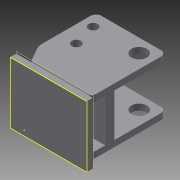
# Autodesk Inventor part: sketss
Saved by Autodesk Inventor 2014 SP2 (Build 180246200, 246)
## iProperties
Created: 2019-06-25
Part Number: sketss
Material: Generic
Document SubType Name: Modeling
Designer: USER PC
Density: 1 g/cm^3
Appearance: Default
Author: USER PC
Autodesk Inventor part; units mm, degrees
ref_plane "YZ Plane" through (0, 0, 0) normal (1, 0, 0) x (0, 1, 0)
ref_plane "XY Plane" through (0, 0, 0) normal (0, 0, 1) x (1, 0, 0)
sketch "Sketch1" plane through (0, 0, 0) normal (0, 0, 1) x (1, 0, 0)
  circle A0 centre (0, 0) radius 15
  circle A1 centre (150, 0) radius 25
  line L0 (-35, 45) -> (-35, -144.3782)
  circle A2 centre (43.934, -106.066) radius 15
  circle A3 centre (20.0962, -75) radius 15
  line L1 (195, 45) -> (-35, 45)
  line L2 (195, -205) -> (0, -205)
  line L3 (195, -205) -> (195, 45)
  line L4 (0, -205) -> (-35, -144.3782)
  line L5 (0, -205) -> (70, -205) construction
  dimension "d22" = 230
  dimension "d23" = 120
  constraints: 12 end point, 4 centre point, 1 coincident, 1 equal length, 1 horizontal, 1 parallel, 1 perpendicular
  measures "d22" distance of L1.start L0.start
  measures "d23" angle of L5 L4
extrude "Extrusion1" add sketch "Sketch1" along normal blind 180
fillet "Fillet1" radius 50 1 edges at (-35, -144.3782, 90)
fillet "Fillet2" radius 20 1 edges at (-35, 45, 90)
fillet "Fillet3" radius 20 1 edges at (195, 45, 90)
fillet "Fillet4" radius 20 1 edges at (195, -205, 90)
fillet "Fillet5" radius 20 1 edges at (0, -205, 90)
sketch "Sketch2" plane through (-35, -130.9808, 0) normal (-1, 0, 0) x (0, 0, 1)
  line L0 (0, 155.9808) -> (180, 155.9808) projected
  line L1 (0, 155.9808) -> (0, 0) projected
  line L2 (180, 155.9808) -> (180, 0) projected
  line L3 (0, 175) -> (0, -75)
  line L4 (0, -75) -> (20, -75)
  line L5 (20, -75) -> (20, -25)
  line L6 (20, -25) -> (160, -25)
  line L7 (160, -25) -> (160, -75)
  line L8 (160, -75) -> (180, -75)
  line L9 (180, -75) -> (180, 175)
  line L10 (180, 175) -> (160, 175)
  line L11 (160, 175) -> (160, 5)
  line L12 (160, 5) -> (20, 5)
  line L13 (20, 5) -> (20, 175)
  line L14 (20, 175) -> (0, 175)
  point P0 (0, 130.9808)
  dimension "d31" = 250
  dimension "d32" = 20
  dimension "d33" = 50
  dimension "d34" = 140
  dimension "d35" = 170
  constraints: 24 end point, 8 parallel, 3 perpendicular, 1 collinear, 1 point on line
  measures "d31" distance of L3.start L3.end
  measures "d32" distance of L3.end L4.end
  measures "d33" distance of L4.end L5.end
  measures "d34" distance of L5.end L6.end
  measures "d35" distance of L10.end L11.end
extrude "Extrusion2" cut sketch "Sketch2" against normal blind 230 contours L3 L14 L13 L0 | L0 L13 L12 L11 L2 L9 L8 L7 L6 L5 L4 L3 L1 | L11 L10 L9 L0 keep common part
sketch "Sketch3" plane through (0, 0, 180) normal (0, 0, 1) x (1, 0, 0)
  circle A0 centre (43.934, -106.066) radius 15 projected
  circle A1 centre (43.934, -106.066) radius 15
  constraints: 1 centre point, 1 coincident, 1 concentric
extrude "Extrusion3" add sketch "Sketch3" against normal blind 20
sketch "Sketch4" plane through (0, 0, 0) normal (0, 0, -1) x (-1, 0, 0)
  circle A0 centre (-43.934, -106.066) radius 15 projected
  circle A1 centre (-43.934, -106.066) radius 15
  constraints: 1 centre point, 1 coincident, 1 concentric
extrude "Extrusion4" add sketch "Sketch4" against normal blind 20
ref_plane "Work Plane1" through (175, -205, 20) normal (0, 1, 0) x (-1, 0, 0)
sketch "Sketch6" plane through (175, -205, 20) normal (0, 1, 0) x (-1, 0, 0)
  line L0 (-19.2308, -36.5385) -> (221.1538, -36.5385)
  line L1 (221.1538, -36.5385) -> (221.1538, 163.4615)
  line L2 (221.1538, 163.4615) -> (-28.8462, 163.4615)
  line L3 (-28.8462, 163.4615) -> (-28.8462, -36.5385)
  line L4 (-28.8462, -36.5385) -> (-19.2308, -36.5385)
  point P0 (175, -20)
  dimension "d55" = 250
  dimension "d56" = 200
  constraints: 10 end point, 2 perpendicular, 1 parallel
  measures "d55" distance between parallel lines of L3 L1
  measures "d56" distance of L0.end L1.end
extrude "Extrusion6" add sketch "Sketch6" against normal blind 20
sketch "Sketch7" plane through (175, -225, 20) normal (0, -1, 0) x (1, 0, 0)
  line L0 (-221.1538, -36.5385) -> (28.8462, -36.5385) projected
  line L1 (28.8462, -36.5385) -> (28.8462, 163.4615) projected
  line L2 (28.8462, 163.4615) -> (-221.1538, 163.4615) projected
  line L3 (-221.1538, 163.4615) -> (-221.1538, -36.5385) projected
  point P0 (-175, -20)
body "Solid1"
